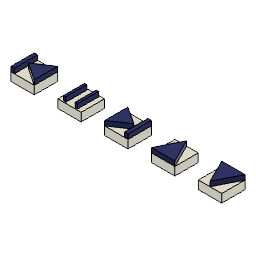
Buttons (Autodesk Fusion 360 design; units mm, degrees)
part number: 2026-06-19-23-47-26-511
Autodesk Fusion 360 part; units mm, degrees
note: some values were not read from the file. Chosen so that the rebuilt part matches the saved one: which bodies a step acts on.
sketch "Sketch1" plane through (0, 0, 0) normal (0, 1, 0) x (1, 0, 0)
  line L0 (109.25, 12.7616) -> (105.5, 15.2616)
  line L1 (109.25, 15.2616) -> (109.75, 15.2616)
  line L2 (95.5, 15.2616) -> (100.5, 15.2616)
  line L3 (90.5, 15.2616) -> (86.75, 12.7616)
  line L4 (109.75, 15.2616) -> (109.75, 10.2616)
  line L5 (86.75, 12.7616) -> (90.5, 10.2616)
  line L6 (97, 15) -> (96.5, 15)
  line L7 (95.5, 10.2616) -> (95.5, 15.2616)
  line L8 (115.5, 15.2616) -> (120.5, 15.2616)
  line L9 (110.5, 10.2616) -> (105.5, 10.2616)
  line L10 (100.5, 10.2616) -> (95.5, 10.2616)
  line L11 (110.5, 15.2616) -> (108, 15.2616)
  line L12 (125.5, 15.2616) -> (130.5, 15.2616)
  line L13 (96.5, 15) -> (96.5, 10.5)
  line L14 (125.5, 10.2616) -> (125.5, 15.2616)
  line L15 (118, 15.2616) -> (120.5, 10.2616)
  line L16 (118, 15.2616) -> (115.5, 10.2616)
  line L17 (97, 15) -> (97, 10.5)
  line L18 (120.5, 10.2616) -> (115.5, 10.2616)
  line L19 (109.25, 12.7616) -> (105.5, 10.2616)
  line L20 (86.25, 15.2616) -> (86.25, 10.2616)
  line L21 (120.5, 15.2616) -> (120.5, 10.2616)
  line L22 (99.5, 15) -> (99, 15)
  line L23 (109.25, 15.2616) -> (109.5, 15.2616)
  line L24 (85.5, 15.2616) -> (90.5, 15.2616)
  line L25 (85.5, 15.2616) -> (86.25, 15.2616)
  line L26 (90.5, 15.2616) -> (90.5, 10.2616)
  line L27 (100.5, 15.2616) -> (100.5, 10.2616)
  line L28 (99.5, 15) -> (99.5, 10.5)
  line L29 (128, 10.2616) -> (125.5, 15.2616)
  line L30 (96.5, 10.5) -> (97, 10.5)
  line L31 (99, 15) -> (99, 10.5)
  line L32 (110.5, 15.2616) -> (110.5, 10.2616)
  line L33 (115.5, 10.2616) -> (115.5, 15.2616)
  line L34 (99, 10.5) -> (99.5, 10.5)
  line L35 (130.5, 15.2616) -> (130.5, 10.2616)
  line L36 (128, 10.2616) -> (130.5, 15.2616)
  line L37 (105.5, 15.2616) -> (110.5, 15.2616)
  line L38 (105.5, 10.2616) -> (105.5, 15.2616)
  line L39 (130.5, 10.2616) -> (125.5, 10.2616)
  line L40 (90.5, 10.2616) -> (85.5, 10.2616)
  line L41 (85.5, 15.2616) -> (85.5, 10.2616)
  dimension "d1" = 5
  dimension "d2" = 5
  dimension "d3" = 5
  dimension "d4" = 5
  dimension "d5" = 5
  dimension "d6" = 5
  dimension "d7" = 5
  dimension "d8" = 5
  dimension "d9" = 5
  dimension "d10" = 5
  dimension "d11" = 0.5
  dimension "d12" = 0.75
  constraint horizontal L24
  constraint vertical L26
  constraint horizontal L40
  constraint horizontal L2
  constraint vertical L27
  constraint horizontal L10
  constraint vertical L7
  constraint horizontal L37
  constraint vertical L32
  constraint horizontal L9
  constraint vertical L38
  constraint horizontal L8
  constraint vertical L21
  constraint horizontal L18
  constraint vertical L33
  constraint horizontal L12
  constraint vertical L35
  constraint horizontal L39
  constraint vertical L14
  constraint perpendicular L40 L41
  constraint midpoint L15.start L8
  constraint midpoint L29.start L39
  constraint midpoint L11.end L37
  constraint midpoint L1.start L11
  constraint coincident L23.end L37
  constraint coincident L4.end L9
  constraint perpendicular L4 L9
  constraint perpendicular L25 L41
  constraint coincident L20.end L40
  constraint perpendicular L20 L40
  constraint perpendicular L6 L7
  constraint perpendicular L27 L34
  constraint perpendicular L28 L34
  constraint perpendicular L13 L30
  constraint perpendicular L17 L30
  constraint perpendicular L31 L34
  constraint collinear L6 L22
  constraint collinear L30 L34
  measures "d1" distance of L3.start L24.start
  measures "d2" distance of L24.start L40.end
  measures "d3" distance of L2.end L2.start
  measures "d4" distance of L7.start L2.start
  measures "d5" distance of L11.start L0.end
  measures "d6" distance of L9.end L0.end
  measures "d7" distance of L8.end L8.start
  measures "d8" distance of L16.end L8.start
  measures "d9" distance of L12.end L12.start
  measures "d10" distance of L12.start L14.start
  measures "d11" distance of L1.end L1.start
  measures "d12" distance of L20.start L24.start
extrude "Extrude1" add sketch "Sketch1" along normal blind 2 contours L0 L19 L38 | L0 L1 L4 L9 L11 L19 L23 L37 | L4 L9 L11 L32 L37 | L2 L7 L10 L27 | L3 L5 L26 | L3 L5 L20 L24 L40 | L20 L24 L25 L40 L41 | L6 L13 L17 L30 | L8 L16 L33 | L8 L15 L21 | L15 L16 L18 | L14 L29 L39 | L12 L29 L36 | L35 L36 L39 | L22 L28 L31 L34 makes body 1 at (118.8333, 0, -11.9283) makes body 2 at (128.8333, 0, -11.9283) makes body 3 at (97.1667, 0, -13.595) makes body 4 at (87.1667, 2, -11.9283) makes body 5 at (107.1667, 0, -13.595)
sketch "Sketch2" plane through (0, 0, 0) normal (0, -1, 0) x (1, 0, 0)
  line L0 (120.5, -10.2616) -> (115.5, -10.2616)
  line L1 (115.5, -10.2616) -> (115.5, -15.2616)
  line L2 (115.5, -15.2616) -> (120.5, -15.2616)
  line L3 (120.5, -15.2616) -> (120.5, -10.2616)
  circle A0 centre (118, -13) radius 0.75
  circle A1 centre (128, -13) radius 0.75
  circle A2 centre (108, -13) radius 0.75
  circle A3 centre (98, -13) radius 0.75
  circle A4 centre (88, -13) radius 0.75
  dimension "d15" = 1.5
  dimension "d16" = 1.5
  dimension "d17" = 1.5
  dimension "d18" = 1.5
  dimension "d19" = 1.5
  measures "d15" diameter of A0
  measures "d16" diameter of A1
  measures "d17" diameter of A2
  measures "d18" diameter of A3
  measures "d19" diameter of A4
extrude "Extrude2" cut sketch "Sketch2" against normal blind 1 contours A0 | A1 | A2 | A3 | A4 bodies 1 2 3 4 5
extrude "Extrude3" add sketch "Sketch1" along normal blind 3 contours L0 L19 L38 | L4 L9 L11 L32 L37 | L3 L5 L26 | L20 L24 L25 L40 L41 | L6 L13 L17 L30 | L15 L16 L18 | L12 L29 L36 | L22 L28 L31 L34 bodies 1 2 3 4 5
extrude "Extrude4" cut sketch "Sketch2" against normal blind 1 contours A0 | A2 bodies 1 5
extrude "Extrude5" cut sketch "Sketch2" against normal blind 1 contours A1 bodies 2
extrude "Extrude6" cut sketch "Sketch2" against normal blind 1 contours A4 bodies 4
extrude "Extrude7" add 1 faces at (89.25, 3, -12.7616) along direction (0, -1, 0) blind 1 separate body on bodies 4 makes body 6
extrude "Extrude8" add 1 faces at (85.75, 3, -13.595) along direction (0, -1, 0) blind 1 separate body on bodies 4 makes body 7
extrude "Extrude9" add 2 faces at (106.75, 3, -12.7616) (110, 3, -13.595) along direction (0, -1, 0) blind 1 separate body on bodies 5 makes body 8 at (106.75, 3, -12.7616) makes body 9 at (109.75, 2.6667, -13.595)
extrude "Extrude10" add 2 faces at (118, 3, -11.9283) (128, 3, -13.595) along direction (0, -1, 0) blind 1 separate body on bodies 1 2 makes body 10 at (118, 3, -11.9283) makes body 11 at (128, 3, -13.595)
extrude "Extrude11" cut 8 faces at (128, 3, -13.595) (118, 3, -11.9283) (106.75, 3, -12.7616) (110, 3, -13.595) (99.1667, 3, -13.5) (96.6667, 3, -13.5) (89.25, 3, -12.7616) (85.75, 3, -13.595) along direction (0, -1, 0) blind 1 on bodies 1 2 3 4 5 bodies 1 2 4 5
extrude "Extrude12" cut 5 faces at (87.9813, 0, -10.9251) (97.9813, 0, -10.9251) (107.9813, 0, -10.9251) (117.9813, 0, -10.9251) (127.9813, 0, -10.9251) along direction (0, 1, 0) blind 0.2 on bodies 1 2 3 4 5 bodies 1 2 3 4 5
extrude "Extrude13" add 5 faces at (88.0913, 1, -13.2327) (97.836, 1, -12.7507) (107.868, 1, -13.1291) (117.836, 1, -12.7507) (127.8031, 1, -13.3522) along direction (0, -1, 0) blind 0.3 separate body on bodies 1 2 3 4 5 makes body 12 at (117.836, 1, -12.7507) makes body 13 at (97.836, 1, -12.7507) makes body 14 at (88.0913, 1, -13.2327) makes body 15 at (107.868, 1, -13.1291) makes body 16 at (127.8031, 1, -13.3522)
